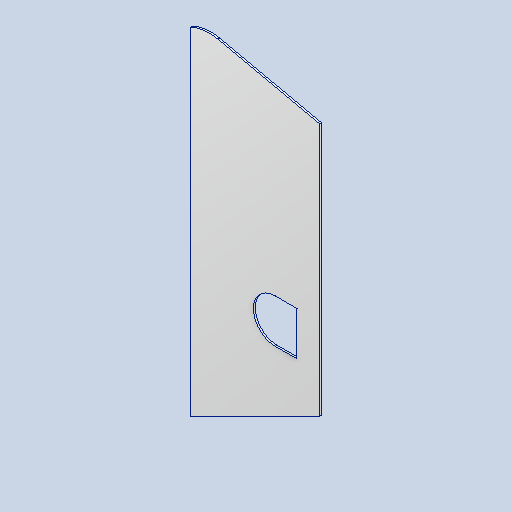
# Autodesk Inventor part: pokrywa prawa
Saved by Autodesk Inventor 2023 (Build 270158000, 158)
## iProperties
Created: 2022-10-11
Part Number: pokrywa prawa
Material: Aluminum 6061
Document SubType Name: Modeling
Designer: komputer
Density: 2.7 g/cm^3
Appearance: Aluminum - Flat
Author: komputer
Autodesk Inventor part; units mm, degrees
ref_plane "YZ Plane" through (0, 0, 0) normal (1, 0, 0) x (0, 1, 0)
ref_plane "XZ Plane" through (0, 0, 0) normal (0, 1, 0) x (-1, 0, 0)
ref_plane "XY Plane" through (0, 0, 0) normal (0, 0, 1) x (1, 0, 0)
sketch "Sketch1" plane through (0, 0, 0) normal (0, 0, 1) x (1, 0, 0)
  line L0 (-17.5, -33.2499) -> (-17.5, 57.9837) projected
  arc A0 (-10.0449, 58.8745) -> (-17.5, 57.9837) centre (-12.5, 47.7794) ccw projected
  line L1 (-10.0449, 58.8745) -> (17.5, 52.7794) projected
  line L2 (17.5, 52.7794) -> (17.5, -15.7501) projected
  line L3 (17.5, -15.7501) -> (-17.5, -33.2499) projected
  line L4 (0.5, 7.1892) -> (0.5, 22.231) projected
  line L5 (0.5, 22.231) -> (-5.8925, 22.231) projected
  line L6 (-5.8925, 22.231) -> (-5.8925, 7.1892) projected
  line L7 (-5.8925, 7.1892) -> (0.5, 7.1892) projected
  point P0 (0, 0)
extrude "Extrusion1" add sketch "Sketch1" along normal blind 0.5 contours L0 A0 L1 L2 L3 | L7 L6 L5 L4
sketch "Sketch2" plane through (0, 0, 0.5) normal (0, 0, 1) x (1, 0, 0)
  circle A0 centre (-7.1425, -8.6154) radius 1.25 projected
  circle A1 centre (-5.3255, 26.728) radius 1.25 projected
  line L0 (7.9908, -12.0691) -> (-3.9853, -13.2144) projected
  line L1 (-3.9853, -13.2144) -> (-3.2796, -20.5939) projected
  line L2 (-3.2796, -20.5939) -> (-5.5333, -16.0863) projected
  line L3 (-5.5333, -16.0863) -> (-14.5107, -20.575) projected
  line L4 (-14.5107, -20.575) -> (-10.0386, -29.5193) projected
  line L5 (-10.0386, -29.5193) -> (-14.6056, -31.8027) projected
  arc A2 (-17.5, -30.0139) -> (-14.6056, -31.8027) centre (-15.5, -30.0139) ccw projected
  line L6 (-17.5, -30.0139) -> (-17.5, -1.8864) projected
  line L7 (-17.5, -1.8864) -> (-7.5, -1.8864) projected
  line L8 (-7.5, -1.8864) -> (-7.5, 7.5751) projected
  line L9 (-7.5, 7.5751) -> (-8.8, 7.5751) projected
  line L10 (-8.8, 26.3195) -> (-8.8, 7.5751) projected
  spline S0 degree 3 poles (-14.2046, 28.2052) (-13.4118, 28.2052) (-12.6544, 28.0226) (-10.9379, 27.4679) (-9.8551, 26.8958) (-8.8077, 26.3237) (-8.8038, 26.3216) (-8.8, 26.3195) knots -0.001308 -0.001308 -0.001308 -0.001308 0.187612 0.187612 0.544344 0.544344 0.545652 0.545652 0.545652 0.545652 projected
  line L11 (-14.2046, 28.2052) -> (-17.5, 28.2052) projected
  line L12 (-17.5, 28.2052) -> (-17.5, 31.9794) projected
  arc A3 (-17.5, 31.9794) -> (-4.376, 33.2499) centre (-12.5, 48.7499) ccw projected
  arc A4 (-4.376, 33.2499) -> (2.7674, 54.4137) centre (-12.5, 47.7794) ccw projected
  arc A5 (3.9006, 55.7887) -> (2.7674, 54.4137) centre (3.6845, 54.8123) ccw projected
  line L13 (3.9006, 55.7887) -> (16.7161, 52.9529) projected
  arc A6 (17.5, 51.9765) -> (16.7161, 52.9529) centre (16.5, 51.9765) ccw projected
  line L14 (17.5, 51.9765) -> (17.5, 12.4999) projected
  line L15 (-17.5, 57.9837) -> (-17.5, -33.2499) projected
  line L16 (-17.5, -33.2499) -> (17.5, -15.7501) projected
  line L17 (17.5, -15.7501) -> (17.5, 52.7794) projected
  line L18 (17.5, 52.7794) -> (-10.0449, 58.8745) projected
  arc A7 (-10.0449, 58.8745) -> (-17.5, 57.9837) centre (-12.5, 47.7794) ccw projected
  line L19 (5.1606, 7.0459) -> (-1.321, 3.6769)
  line L20 (4.7678, -6.2957) -> (11.3303, -6.2957)
  line L21 (11.3303, -6.2957) -> (11.3303, 7.0459)
  circle A8 centre (5.4296, 0.5354) radius 5.9007
  line L22 (5.4296, 0.5354) -> (11.3303, 0.5354)
  line L23 (11.3303, 0.5354) -> (11.3303, 6.4362)
  line L24 (11.3303, 6.4362) -> (5.4296, 6.4362)
  line L25 (5.4296, 6.4362) -> (5.4296, 0.5354)
  line L26 (11.3303, 0.5354) -> (5.4296, 0.5354)
  line L27 (5.4296, 0.5354) -> (5.4296, -5.3653)
  line L28 (5.4296, -5.3653) -> (11.3303, -5.3653)
  line L29 (11.3303, -5.3653) -> (11.3303, 0.5354)
  line L30 (17.5, 12.4999) -> (17.5, -15.0638) projected
  arc A9 (6.7111, 29.0491) -> (5.9939, 27.4054) centre (10.3942, 26.4637) ccw projected
  line L31 (17.5, -15.0638) -> (8.7236, -19.7311) projected
  line L32 (8.7236, -19.7311) -> (7.9908, -12.0691) projected
  arc A10 (11.3142, 37.9135) -> (11.9006, 39.3324) centre (2.3926, 42.4306) ccw projected
  line L33 (11.3142, 37.9135) -> (7.448, 30.2774) projected
  arc A11 (6.7111, 29.0491) -> (7.448, 30.2774) centre (-1.4736, 34.7946) ccw projected
  line L34 (5.9939, 27.4054) -> (-3.5211, -6.2541) projected
  arc A12 (-3.5211, -6.2541) -> (-3.1362, -6.7629) centre (-3.1362, -6.3629) ccw projected
  line L35 (-3.1362, -6.7629) -> (10.9647, -6.7629) projected
  arc A13 (10.9647, -6.7629) -> (11.3638, -6.3887) centre (10.9647, -6.3629) ccw projected
  line L36 (11.3638, -6.3887) -> (14.294, 38.9522) projected
  arc A14 (14.294, 38.9522) -> (11.9006, 39.3324) centre (13.0671, 38.9522) ccw projected
  point P0 (0, 0)
  point P1 (17.5, 7.0459)
  point P2 (4.8837, -6.7629)
  constraints: 22 end point, 4 parallel, 3 horizontal, 2 perpendicular, 2 point on line, 1 vertical, 4 other
extrude "Extrusion2" cut sketch "Sketch2" against normal blind 10 contours L28 A8 L21 | A8 L24 L21 | L22 L25 A8 | A8 L27 L22 | A8 L25 L27
body "Solid1"
